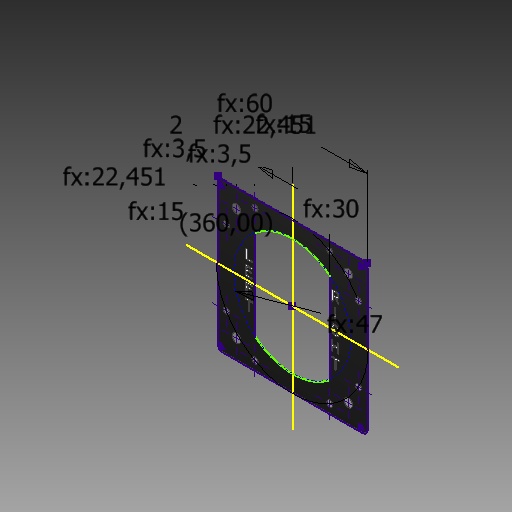
# Autodesk Inventor part: FrontMask
Saved by Autodesk Inventor 2019 (Build 230136000, 136)
## iProperties
Created: 2018-04-27
Part Number: FrontMask
Material: Generic
Document SubType Name: Modeling
Designer: Fierl
Density: 1 g/cm^3
Appearance: Default
Mass: 0.201646 g
Surface Area: 40.8113 cm^2
Volume: 0.201646 cm^3
Author: Fierl
Autodesk Inventor part; units mm, degrees
ref_plane "YZ Plane" through (0, 0, 0) normal (1, 0, 0) x (0, 1, 0)
ref_plane "XZ Plane" through (0, 0, 0) normal (0, 1, 0) x (-1, 0, 0)
ref_plane "XY Plane" through (0, 0, 0) normal (0, 0, 1) x (1, 0, 0)
sketch "Sketch1" plane through (0, 0, 0) normal (0, 0, 1) x (1, 0, 0)
  line L0 (0, -42.5799) -> (0, 42.5799) projected
  line L1 (-42.5799, 0) -> (42.5799, 0) projected
  line L2 (-28, 30) -> (28, 30)
  line L3 (30, 28) -> (30, -28)
  line L4 (28, -30) -> (-28, -30)
  line L5 (-30, -28) -> (-30, 28)
  arc A0 (-28, 30) -> (-30, 28) centre (-28, 28) ccw
  arc A1 (30, 28) -> (28, 30) centre (28, 28) ccw
  arc A2 (28, -30) -> (30, -28) centre (28, -28) ccw
  arc A3 (-30, -28) -> (-28, -30) centre (-28, -28) ccw
  circle A4 centre (0, 0) radius 23.5 construction
  line L6 (15, -18.0901) -> (15, 18.0901)
  line L7 (-15, 18.0901) -> (-15, -18.0901)
  arc A5 (-15, -18.0901) -> (15, -18.0901) centre (0, 0) ccw
  arc A6 (15, 18.0901) -> (-15, 18.0901) centre (0, 0) ccw
  line L8 (-20.0247, 10.8439) -> (-14.5804, 10.8439) construction
  line L9 (-14.5804, 10.8439) -> (-14.5804, -13.9369) construction
  line L10 (-14.5804, -13.9369) -> (-20.0247, -13.9369) construction
  line L11 (-20.0247, -13.9369) -> (-20.0247, 10.8439) construction
  line L12 (15.4141, 13.7154) -> (19.2359, 13.7154) construction
  line L13 (19.2359, 13.7154) -> (19.2359, -13.6884) construction
  line L14 (19.2359, -13.6884) -> (15.4141, -13.6884) construction
  line L15 (15.4141, -13.6884) -> (15.4141, 13.7154) construction
  line L16 (-16.2504, 6.9023) -> (-18.6282, 6.9023)
  line L17 (-18.6282, 6.9023) -> (-18.6282, 10.5951)
  spline S0 degree 2 poles (-18.6282, 10.5951) (-18.6282, 10.8439) (-18.3917, 10.8439) knots 0 0 0 1 1 1
  spline S1 degree 2 poles (-18.3917, 10.8439) (-18.1582, 10.8439) (-18.1582, 10.5951) knots 0 0 0 1 1 1
  line L18 (-18.1582, 10.5951) -> (-18.1582, 7.3846)
  line L19 (-18.1582, 7.3846) -> (-16.2504, 7.3846)
  spline S2 degree 2 poles (-16.2504, 7.3846) (-16.0107, 7.3846) (-16.0107, 7.145) knots 0 0 0 1 1 1
  spline S3 degree 2 poles (-16.0107, 7.145) (-16.0107, 6.9023) (-16.2504, 6.9023) knots 0 0 0 1 1 1
  line L20 (-16.3318, 1.102) -> (-18.7097, 1.102)
  line L21 (-18.7097, 1.102) -> (-18.7097, 5.0375)
  line L22 (-18.7097, 5.0375) -> (-16.3318, 5.0375)
  spline S4 degree 2 poles (-16.3318, 5.0375) (-16.0921, 5.0375) (-16.0921, 4.7948) knots 0 0 0 1 1 1
  spline S5 degree 2 poles (-16.0921, 4.7948) (-16.0921, 4.5491) (-16.3318, 4.5491) knots 0 0 0 1 1 1
  line L23 (-16.3318, 4.5491) -> (-18.2396, 4.5491)
  line L24 (-18.2396, 4.5491) -> (-18.2396, 3.5045)
  line L25 (-18.2396, 3.5045) -> (-16.4485, 3.5045)
  spline S6 degree 2 poles (-16.4485, 3.5045) (-16.2089, 3.5045) (-16.2089, 3.2618) knots 0 0 0 1 1 1
  spline S7 degree 2 poles (-16.2089, 3.2618) (-16.2089, 3.016) (-16.4485, 3.016) knots 0 0 0 1 1 1
  line L26 (-16.4485, 3.016) -> (-18.2396, 3.016)
  line L27 (-18.2396, 3.016) -> (-18.2396, 1.5905)
  line L28 (-18.2396, 1.5905) -> (-16.3318, 1.5905)
  spline S8 degree 2 poles (-16.3318, 1.5905) (-16.0921, 1.5905) (-16.0921, 1.3478) knots 0 0 0 1 1 1
  spline S9 degree 2 poles (-16.0921, 1.3478) (-16.0921, 1.102) (-16.3318, 1.102) knots 0 0 0 1 1 1
  line L29 (-16.2888, -1.2604) -> (-18.1966, -1.2604)
  line L30 (-18.1966, -1.2604) -> (-18.1966, -2.3019)
  line L31 (-18.1966, -2.3019) -> (-16.7373, -2.3019)
  spline S10 degree 2 poles (-16.7373, -2.3019) (-16.4977, -2.3019) (-16.4977, -2.5446) knots 0 0 0 1 1 1
  spline S11 degree 2 poles (-16.4977, -2.5446) (-16.4977, -2.7904) (-16.7373, -2.7904) knots 0 0 0 1 1 1
  line L32 (-16.7373, -2.7904) -> (-18.1966, -2.7904)
  line L33 (-18.1966, -2.7904) -> (-18.1966, -4.4955)
  spline S12 degree 2 poles (-18.1966, -4.4955) (-18.1966, -4.7443) (-18.4301, -4.7443) knots 0 0 0 1 1 1
  spline S13 degree 2 poles (-18.4301, -4.7443) (-18.6666, -4.7443) (-18.6666, -4.4955) knots 0 0 0 1 1 1
  line L34 (-18.6666, -4.4955) -> (-18.6666, -0.772)
  line L35 (-18.6666, -0.772) -> (-16.2888, -0.772)
  spline S14 degree 2 poles (-16.2888, -0.772) (-16.0491, -0.772) (-16.0491, -1.0147) knots 0 0 0 1 1 1
  spline S15 degree 2 poles (-16.0491, -1.0147) (-16.0491, -1.2604) (-16.2888, -1.2604) knots 0 0 0 1 1 1
  line L36 (-16.0752, -7.0883) -> (-17.1044, -7.0883)
  line L37 (-17.1044, -7.0883) -> (-17.1044, -10.4954)
  spline S16 degree 2 poles (-17.1044, -10.4954) (-17.1044, -10.7565) (-17.3533, -10.7565) knots 0 0 0 1 1 1
  spline S17 degree 2 poles (-17.3533, -10.7565) (-17.6052, -10.7565) (-17.6052, -10.4954) knots 0 0 0 1 1 1
  line L38 (-17.6052, -10.4954) -> (-17.6052, -7.0883)
  line L39 (-17.6052, -7.0883) -> (-18.6344, -7.0883)
  spline S18 degree 2 poles (-18.6344, -7.0883) (-18.8894, -7.0883) (-18.8894, -6.8303) knots 0 0 0 1 1 1
  spline S19 degree 2 poles (-18.8894, -6.8303) (-18.8894, -6.5753) (-18.6344, -6.5753) knots 0 0 0 1 1 1
  line L40 (-18.6344, -6.5753) -> (-16.0752, -6.5753)
  spline S20 degree 2 poles (-16.0752, -6.5753) (-15.8172, -6.5753) (-15.8172, -6.8303) knots 0 0 0 1 1 1
  spline S21 degree 2 poles (-15.8172, -6.8303) (-15.8172, -7.0883) (-16.0752, -7.0883) knots 0 0 0 1 1 1
  spline S22 degree 2 poles (18.6875, 12.5695) (18.6875, 11.9643) (18.2912, 11.6601) knots 0 0 0 1 1 1
  spline S23 degree 2 poles (18.2912, 11.6601) (18.0301, 11.4635) (17.769, 11.4635) knots 0 0 0 1 1 1
  line L41 (17.769, 11.4635) -> (17.7106, 11.4604)
  line L42 (17.7106, 11.4604) -> (18.6415, 10.1271)
  spline S24 degree 2 poles (18.6415, 10.1271) (18.6875, 10.0565) (18.6875, 9.9796) knots 0 0 0 1 1 1
  spline S25 degree 2 poles (18.6875, 9.9796) (18.6875, 9.8813) (18.537, 9.7308) (18.4448, 9.7308) knots 0 0 0 1 2 2 2
  spline S26 degree 2 poles (18.4448, 9.7308) (18.3342, 9.7308) (18.2636, 9.8353) knots 0 0 0 1 1 1
  line L43 (18.2636, 9.8353) -> (17.1177, 11.4635)
  line L44 (17.1177, 11.4635) -> (16.3558, 11.4635)
  line L45 (16.3558, 11.4635) -> (16.3558, 9.9796)
  spline S27 degree 2 poles (16.3558, 9.9796) (16.3558, 9.7308) (16.1192, 9.7308) knots 0 0 0 1 1 1
  spline S28 degree 2 poles (16.1192, 9.7308) (15.8796, 9.7308) (15.8796, 9.9796) knots 0 0 0 1 1 1
  line L46 (15.8796, 9.9796) -> (15.8796, 13.7154)
  line L47 (15.8796, 13.7154) -> (17.5601, 13.7154)
  spline S29 degree 2 poles (17.5601, 13.7154) (18.0178, 13.7154) (18.3435, 13.4174) knots 0 0 0 1 1 1
  spline S30 degree 2 poles (18.3435, 13.4174) (18.6875, 13.0918) (18.6875, 12.5695) knots 0 0 0 1 1 1
  spline S31 degree 2 poles (18.2175, 12.5695) (18.2175, 12.8767) (18.0209, 13.0641) knots 0 0 0 1 1 1
  spline S32 degree 2 poles (18.0209, 13.0641) (17.8335, 13.2331) (17.5601, 13.2331) knots 0 0 0 1 1 1
  line L48 (17.5601, 13.2331) -> (16.3558, 13.2331)
  line L49 (16.3558, 13.2331) -> (16.3558, 11.952)
  line L50 (16.3558, 11.952) -> (17.769, 11.952)
  spline S33 degree 2 poles (17.769, 11.952) (17.898, 11.952) (18.0301, 12.0749) knots 0 0 0 1 1 1
  spline S34 degree 2 poles (18.0301, 12.0749) (18.2175, 12.2439) (18.2175, 12.5695) knots 0 0 0 1 1 1
  spline S35 degree 2 poles (17.3803, 4.1732) (17.3803, 3.9244) (17.1438, 3.9244) knots 0 0 0 1 1 1
  spline S36 degree 2 poles (17.1438, 3.9244) (16.9041, 3.9244) (16.9041, 4.1732) knots 0 0 0 1 1 1
  line L51 (16.9041, 4.1732) -> (16.9041, 7.6694)
  spline S37 degree 2 poles (16.9041, 7.6694) (16.9041, 7.9121) (17.1438, 7.9121) knots 0 0 0 1 1 1
  spline S38 degree 2 poles (17.1438, 7.9121) (17.3803, 7.9121) (17.3803, 7.6694) knots 0 0 0 1 1 1
  line L52 (17.3803, 7.6694) -> (17.3803, 4.1732)
  spline S39 degree 2 poles (18.4925, -0.4473) (18.4925, -1.2491) (18.0562, -1.6393) knots 0 0 0 1 1 1
  spline S40 degree 2 poles (18.0562, -1.6393) (17.749, -1.9127) (17.3404, -1.9127) knots 0 0 0 1 1 1
  spline S41 degree 2 poles (17.3404, -1.9127) (16.643, -1.9127) (16.1822, -1.2676) knots 0 0 0 1 1 1
  spline S42 degree 2 poles (16.1822, -1.2676) (15.7582, -0.6808) (15.7582, 0.0842) knots 0 0 0 1 1 1
  spline S43 degree 2 poles (15.7582, 0.0842) (15.7582, 1.0181) (16.2006, 1.5896) knots 0 0 0 1 1 1
  spline S44 degree 2 poles (16.2006, 1.5896) (16.6184, 2.1426) (17.2759, 2.1426) knots 0 0 0 1 1 1
  spline S45 degree 2 poles (17.2759, 2.1426) (17.7367, 2.1426) (18.0132, 1.9521) knots 0 0 0 1 1 1
  spline S46 degree 2 poles (18.0132, 1.9521) (18.1791, 1.8415) (18.3696, 1.5496) knots 0 0 0 1 1 1
  spline S47 degree 2 poles (18.3696, 1.5496) (18.4218, 1.4728) (18.4218, 1.3929) knots 0 0 0 1 1 1
  spline S48 degree 2 poles (18.4218, 1.3929) (18.4218, 1.2977) (18.2774, 1.1656) (18.1822, 1.1656) knots 0 0 0 1 2 2 2
  spline S49 degree 2 poles (18.1822, 1.1656) (18.0624, 1.1656) (17.9794, 1.2762) knots 0 0 0 1 1 1
  spline S50 degree 2 poles (17.9794, 1.2762) (17.835, 1.479) (17.7367, 1.5435) knots 0 0 0 1 1 1
  spline S51 degree 2 poles (17.7367, 1.5435) (17.5739, 1.6541) (17.2759, 1.6541) knots 0 0 0 1 1 1
  spline S52 degree 2 poles (17.2759, 1.6541) (16.8058, 1.6541) (16.2344, 0.7877) (16.2344, 0.0842) knots 0 0 0 1 2 2 2
  spline S53 degree 2 poles (16.2344, 0.0842) (16.2344, -0.4872) (16.5201, -0.9296) knots 0 0 0 1 1 1
  spline S54 degree 2 poles (16.5201, -0.9296) (16.8396, -1.4243) (17.3404, -1.4243) knots 0 0 0 1 1 1
  spline S55 degree 2 poles (17.3404, -1.4243) (17.7828, -1.4243) (17.921, -0.9942) knots 0 0 0 1 1 1
  spline S56 degree 2 poles (17.921, -0.9942) (17.9978, -0.773) (17.9978, -0.306) knots 0 0 0 1 1 1
  line L53 (17.9978, -0.306) -> (17.4694, -0.306)
  spline S57 degree 2 poles (17.4694, -0.306) (17.2236, -0.306) (17.2236, -0.0602) knots 0 0 0 1 1 1
  spline S58 degree 2 poles (17.2236, -0.0602) (17.2236, 0.1825) (17.4694, 0.1825) knots 0 0 0 1 1 1
  line L54 (17.4694, 0.1825) -> (18.4925, 0.1825)
  line L55 (18.4925, 0.1825) -> (18.4925, -0.4473)
  spline S59 degree 2 poles (18.5339, -7.4427) (18.5339, -7.6884) (18.3005, -7.6884) knots 0 0 0 1 1 1
  spline S60 degree 2 poles (18.3005, -7.6884) (18.0639, -7.6884) (18.0639, -7.4427) knots 0 0 0 1 1 1
  line L56 (18.0639, -7.4427) -> (18.0639, -5.8328)
  line L57 (18.0639, -5.8328) -> (16.2882, -5.8328)
  line L58 (16.2882, -5.8328) -> (16.2882, -7.4427)
  spline S61 degree 2 poles (16.2882, -7.4427) (16.2882, -7.6884) (16.0547, -7.6884) knots 0 0 0 1 1 1
  spline S62 degree 2 poles (16.0547, -7.6884) (15.8181, -7.6884) (15.8181, -7.4427) knots 0 0 0 1 1 1
  line L59 (15.8181, -7.4427) -> (15.8181, -3.9496)
  spline S63 degree 2 poles (15.8181, -3.9496) (15.8181, -3.7038) (16.0547, -3.7038) knots 0 0 0 1 1 1
  spline S64 degree 2 poles (16.0547, -3.7038) (16.2882, -3.7038) (16.2882, -3.9496) knots 0 0 0 1 1 1
  line L60 (16.2882, -3.9496) -> (16.2882, -5.3443)
  line L61 (16.2882, -5.3443) -> (18.0639, -5.3443)
  line L62 (18.0639, -5.3443) -> (18.0639, -3.9496)
  spline S65 degree 2 poles (18.0639, -3.9496) (18.0639, -3.7038) (18.3005, -3.7038) knots 0 0 0 1 1 1
  spline S66 degree 2 poles (18.3005, -3.7038) (18.5339, -3.7038) (18.5339, -3.9496) knots 0 0 0 1 1 1
  line L63 (18.5339, -3.9496) -> (18.5339, -7.4427)
  line L64 (18.5524, -10.0202) -> (17.5232, -10.0202)
  line L65 (17.5232, -10.0202) -> (17.5232, -13.4273)
  spline S67 degree 2 poles (17.5232, -13.4273) (17.5232, -13.6884) (17.2743, -13.6884) knots 0 0 0 1 1 1
  spline S68 degree 2 poles (17.2743, -13.6884) (17.0224, -13.6884) (17.0224, -13.4273) knots 0 0 0 1 1 1
  line L66 (17.0224, -13.4273) -> (17.0224, -10.0202)
  line L67 (17.0224, -10.0202) -> (15.9932, -10.0202)
  spline S69 degree 2 poles (15.9932, -10.0202) (15.7382, -10.0202) (15.7382, -9.7621) knots 0 0 0 1 1 1
  spline S70 degree 2 poles (15.7382, -9.7621) (15.7382, -9.5071) (15.9932, -9.5071) knots 0 0 0 1 1 1
  line L68 (15.9932, -9.5071) -> (18.5524, -9.5071)
  spline S71 degree 2 poles (18.5524, -9.5071) (18.8104, -9.5071) (18.8104, -9.7621) knots 0 0 0 1 1 1
  spline S72 degree 2 poles (18.8104, -9.7621) (18.8104, -10.0202) (18.5524, -10.0202) knots 0 0 0 1 1 1
  point P0 (-30, 30)
  point P1 (30, 30)
  point P2 (-22.4506, 22.4506)
  point P3 (-26.5, 15)
  point P4 (-15, 26.5)
  point P5 (-15, -26.5)
  point P6 (-22.4506, -22.4506)
  point P7 (-26.5, -15)
  point P8 (26.5, -15)
  point P9 (22.4506, -22.4506)
  point P10 (15, -26.5)
  point P11 (15, 26.5)
  point P12 (22.4506, 22.4506)
  point P13 (26.5, 15)
  dimension "screw_distance_center" = 15
  dimension "d0" = 60
  dimension "d1" = 2
  dimension "d2" = 22.4506
  dimension "d3" = 22.4506
  dimension "d4" = 15
  dimension "d5" = 15
  dimension "d6" = 3.5
  dimension "d7" = 3.5
  dimension "d10" = 360
  dimension "d28" = 47
  dimension "d29" = 30
  constraints: 16 point on circle, 12 end point, 8 tangent, 7 centre point, 4 parallel, 4 point on line, 3 equal radius, 2 perpendicular, 1 coincident, 1 horizontal, 20 other
  measures "d0" distance of point (-30, 30) point (30, 30)
  measures "d1" radius of A0
  measures "d2" distance from line of L0 point (-22.451, 22.451)
  measures "d3" distance from line of L1 point (-22.451, 22.451)
  measures "d4" distance from line of L1 point (-26.5, 15)
  measures "d5" distance from line of L0 point (-15, 26.5)
  measures "d6" distance from line of L2 point (-15, 26.5)
  measures "d7" distance from line of L5 point (-26.5, 15)
  measures "d28" diameter of A4
  measures "d29" distance between parallel lines of L6 L7
extrude "Extrusion1" add sketch "Sketch1" against normal blind 0.1 contours L4 A3 L5 L1 L7 A5 L0 | L0 A5 L6 L1 S42 S41 S40 S39 L55 L3 A2 L4 | A5 L7 L1 L0 | L0 L1 L6 A5 | L1 L7 A6 L0 | L0 A6 L6 L1 | A6 L7 L1 L5 A0 L2 L0 | L0 L2 A1 L3 L1 L55 L54 S58 S53 S52 S51 S50 S49 S48 S47 S46 S45 S44 S43 S42 L6 A6 | S42 S43 S44 S45 S46 S47 S48 S49 S50 S51 S52 S53 L1 | L1 S53 S54 S55 S56 L53 S57 S58 L55 S39 S40 S41 S42 | L1 S58 L54 L55 | L1 S58 S57 L53 S56 S55 S54 S53 | L16 L17 S0 S1 L18 L19 S2 S3 | L20 L21 L22 S4 S5 L23 L24 L25 S6 S7 L26 L27 L28 S8 S9 | L29 L30 L31 S10 S11 L32 L33 S12 S13 L34 L35 S14 S15 | L36 L37 S16 S17 L38 L39 S18 S19 L40 S20 S21 | S22 S23 L41 L42 S24 S25 S26 L43 L44 L45 S27 S28 L46 L47 S29 S30 | S34 S33 L50 L49 L48 S32 S31 | S35 S36 L51 S37 S38 L52 | S59 S60 L56 L57 L58 S61 S62 L59 S63 S64 L60 L61 L62 S65 S66 L63 | L64 L65 S67 S68 L66 L67 S69 S70 L68 S71 S72
hole "Hole1" at (-22.4506, 22.4506, 0) at (22.4506, 22.4506, 0) at (22.4506, -22.4506, 0) at (-22.4506, -22.4506, 0) direction (0, 0, -1) diameter 3.4 end through all clearance for "Countersunk Flat Head Screw DIN EN ISO 2009" size "M3" standard "DIN"
hole "Hole2" at (-26.5, 15, 0) at (-15, 26.5, 0) at (-15, -26.5, 0) at (-26.5, -15, 0) at (26.5, -15, 0) at (15, -26.5, 0) at (15, 26.5, 0) at (26.5, 15, 0) direction (0, 0, -1) diameter 2.4 end through all clearance for "Countersunk Flat Head Screw DIN EN ISO 2009" size "M2" standard "DIN"
extrude "Extrusion2" cut sketch "Sketch1" against normal blind 1 contours A5 L7 L1 L0 | L0 L1 L6 A5 | L1 L7 A6 L0 | L0 A6 L6 L1
extrude "Extrusion3" cut sketch "Sketch1" against normal blind 0.05 contours S42 S43 S44 S45 S46 S47 S48 S49 S50 S51 S52 S53 L1 | L1 S53 S54 S55 S56 L53 S57 S58 L55 S39 S40 S41 S42 | L1 S58 L54 L55 | L16 L17 S0 S1 L18 L19 S2 S3 | L20 L21 L22 S4 S5 L23 L24 L25 S6 S7 L26 L27 L28 S8 S9 | L29 L30 L31 S10 S11 L32 L33 S12 S13 L34 L35 S14 S15 | L36 L37 S16 S17 L38 L39 S18 S19 L40 S20 S21 | S22 S23 L41 L42 S24 S25 S26 L43 L44 L45 S27 S28 L46 L47 S29 S30 | S35 S36 L51 S37 S38 L52 | S59 S60 L56 L57 L58 S61 S62 L59 S63 S64 L60 L61 L62 S65 S66 L63 | L64 L65 S67 S68 L66 L67 S69 S70 L68 S71 S72
equation "\"screw_distance_center\" = 15"
equation "\"d0\" = backplate_width"
equation "\"d2\" = hole_distance"
equation "\"d3\" = hole_distance"
equation "\"d4\" = screw_distance_center"
equation "\"d5\" = screw_distance_center"
equation "\"d6\" = screw_distance_outside"
equation "\"d7\" = screw_distance_outside"
equation "\"d28\" = circle_dimension_inner"
equation "\"d29\" = mask_width"
equation "\"encoder_axis\" = 8"
equation "\"encoder_emboss\" = 0"
equation "\"encoders\" = 0"
equation "\"encoder_width\" = 27"
equation "\"front_plate_thickness\" = 2"
equation "\"glass_thickness\" = 2"
equation "\"screw_distance_outside\" = 3.5"
equation "\"encoder_rad\" = 49"
equation "\"encoder_extrude_hight\" = 3"
equation "\"ring_top_thickness\" = 2"
equation "\"ring_outer_bevel_depth\" = 0.5"
equation "\"ring_depth\" = 6"
equation "\"ring_outer_bevel_height\" = 3"
equation "\"ring_inner_bevel_depth\" = 3.5"
equation "\"ring_thickness\" = 9"
equation "\"hole_from_center\" = 63.5"
equation "\"circle_dimension_inner\" = 47"
equation "\"circle_dimension\" = 56"
equation "\"backplate_width\" = 60"
equation "\"hole_distance\" = 22.45064"
equation "\"mask_width\" = 30"
equation "\"pointer_axis\" = 1"
equation "\"pointer_axis_outside\" = 3"
equation "\"pointer_length\" = 18"
body "Solid1"
